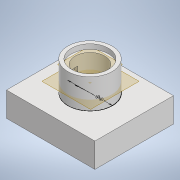
# Autodesk Inventor part: BrakeCover
Saved by Autodesk Inventor 2021 (Build 250183000, 183)
## iProperties
Created: 2021-03-19
Part Number: BrakeCover
Material: Generic
Document SubType Name: Modeling
Designer: ben
Density: 1 g/cm^3
Appearance: Default
Author: ben
Autodesk Inventor part; units mm, degrees
ref_plane "YZ Plane" through (0, 0, 0) normal (1, 0, 0) x (0, 1, 0)
ref_plane "XZ Plane" through (0, 0, 0) normal (0, 1, 0) x (-1, 0, 0)
ref_plane "XY Plane" through (0, 0, 0) normal (0, 0, 1) x (1, 0, 0)
sketch "Sketch2" plane through (0, 0, 0) normal (0, 1, 0) x (-1, 0, 0)
  line L0 (90, -80) -> (-90, -80)
  line L1 (-90, -80) -> (-90, 80)
  line L2 (-90, 80) -> (90, 80)
  line L3 (90, 80) -> (90, -80)
  line L4 (90, -80) -> (-90, 80) construction
  line L5 (-90, -80) -> (90, 80) construction
  point P0 (0, 0)
  dimension "d0" = 180
  dimension "d1" = 160
  constraints: 12 end point, 2 midpoint, 2 parallel, 1 horizontal, 1 perpendicular
  measures "d0" distance of L1.end L2.end
  measures "d1" distance of L0.end L1.end
extrude "Extrusion1" add sketch "Sketch2" along normal blind 50
shell "Shell1" thickness 10 removed faces 1 at (30, 0, -26.6667)
sketch "Sketch4" plane through (0, 0, 0) normal (0, -1, 0) x (1, 0, 0)
  line L0 (-80, 70) -> (80, 70) projected
  line L1 (-80, -70) -> (-80, 70) projected
  line L2 (80, -70) -> (-80, -70) projected
  line L3 (80, 70) -> (80, -70) projected
  point P0 (0, 0)
extrude "Extrusion3" add sketch "Sketch4" against normal blind 10 separate body
sketch "Sketch5" plane through (0, 50, 0) normal (0, 1, 0) x (1, 0, 0)
  circle A0 centre (0, 0) radius 30
  circle A1 centre (0, 0) radius 45
  dimension "d9" = 60
  dimension "d10" = 90
  constraints: 2 centre point, 2 coincident
  measures "d9" diameter of A0
  measures "d10" diameter of A1
extrude "Extrusion4" add sketch "Sketch5" along normal blind 60 separate body
extrude "Extrusion5" cut sketch "Sketch5" against normal blind 120 contours A0 bodies 1
ref_plane "Work Plane1" through (0, 100, 0) normal (0, 1, 0) x (1, 0, 0)
sketch "Sketch6" plane through (0, 110, 0) normal (0, 1, 0) x (1, 0, 0)
  circle A0 centre (0, 0) radius 30 projected
  circle A1 centre (0, 0) radius 37.5
  dimension "d16" = 75
  constraints: 1 centre point, 1 coincident
  measures "d16" diameter of A1
extrude "Extrusion6" cut sketch "Sketch6" against normal blind 10 bodies 3
ref_plane "Work Plane2" through (0, 70, 0) normal (0, 1, 0) x (1, 0, 0)
sketch "Sketch8" plane through (0, 70, 0) normal (0, 1, 0) x (1, 0, 0)
  circle A0 centre (0, 0) radius 37.5 projected
  circle A1 centre (0, 0) radius 30 projected
  line L0 (0, 0) -> (29.5442, -5.2094)
  circle A2 centre (0, 0) radius 30 projected
  line L1 (0, 0) -> (30, 0) construction
  line L2 (29.5442, -5.2094) -> (36.9303, -6.5118)
  line L3 (0, 0) -> (-30, 0)
  circle A3 centre (0, 0) radius 30 projected
  line L4 (-30, 0) -> (-30, 5)
  line L5 (-30, 5) -> (-37.5, 5)
  line L6 (-37.5, 5) -> (-37.5, 0)
  line L7 (-37.5, 0) -> (-30, 0)
  line L8 (29.5442, -5.2094) -> (36.9303, -6.5118)
  line L9 (36.9303, -6.5118) -> (37.7985, -1.5878)
  line L10 (37.7985, -1.5878) -> (30.4125, -0.2854)
  line L11 (30.4125, -0.2854) -> (29.5442, -5.2094)
  arc A4 (-30, 0) -> (29.5442, -5.2094) centre (0, 0) ccw
  arc A5 (-37.5, 0) -> (36.9303, -6.5118) centre (0, 0) ccw
  line L12 (-30, 5) -> (-29.5804, 5)
  line L13 (30.4125, -0.2854) -> (29.9992, -0.2125)
  point P0 (37.4688, -1.5296)
  point P1 (-37.1652, 5)
  dimension "d20" = 10
  dimension "d21" = 5
  dimension "d22" = 5
  constraints: 28 end point, 7 point on circle, 4 parallel, 3 horizontal, 2 centre point, 2 perpendicular, 2 tangent, 2 vertical, 1 coincident, 1 equal length, 4 other
  measures "d20" angle of L0 L1
  measures "d21" distance of L3.end L4.end
  measures "d22" distance of L9.end L2.end
extrude "Extrusion7" cut sketch "Sketch8" along normal blind 10 contours L7 A1 L2 A0 | A0 L5 L4 L7 | L2 L11 L10 A0 | L4 L12 A1 | A1 L13 L11 bodies 3
sketch "Sketch9" plane through (0, 100, 0) normal (0, 1, 0) x (1, 0, 0)
  line L0 (37.4688, -1.5296) -> (29.9992, -0.2125) projected
  arc A0 (-29.5804, 5) -> (29.9992, -0.2125) centre (0, 0) ccw projected
  line L1 (-29.5804, 5) -> (-37.1652, 5) projected
  arc A1 (-37.1652, 5) -> (37.4688, -1.5296) centre (0, 0) ccw projected
  line L2 (29.9992, -0.2125) -> (37.4688, -1.5296)
  line L3 (37.4688, -1.5296) -> (35.7323, -11.3777)
  line L4 (35.7323, -11.3777) -> (28.2628, -10.0606)
  line L5 (28.2628, -10.0606) -> (29.9992, -0.2125)
  line L6 (35.7323, -11.3777) -> (35.7323, -11.3777)
  circle A2 centre (0, 0) radius 37.5 projected
  point P0 (36.9303, -6.5118)
  point P1 (28.2628, -10.0606)
  dimension "d25" = 10
  constraints: 10 end point, 2 parallel, 1 perpendicular, 1 point on circle
  measures "d25" distance of L0.start L3.end
extrude "Extrusion9" cut sketch "Sketch9" against normal up to surface (30 mm away) contours L3 L4 A0 L0 | A1 L3 bodies 3
